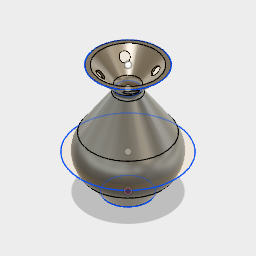
huaping (Autodesk Fusion 360 design; units mm, degrees)
Autodesk Fusion 360 part; units mm, degrees
sketch "草图1" plane through (0, 0, 0) normal (0, 1, 0) x (1, 0, 0)
  circle A0 centre (0, 0) radius 14.1421
  circle A1 through (34.6774, 0, 25) (-17.3387, 30.0315, 25) (-17.3387, -30.0315, 25)
  circle A2 through (7.0711, 0, 65) (-3.5355, 6.1237, 65) (-3.5355, -6.1237, 65)
  circle A3 through (22.3607, 0, 80) (-11.1803, 19.3649, 80) (-11.1803, -19.3649, 80)
loft "放样1" add profiles "草图1", "草图1" section 1 section 2 contours A1 in plane through (0, 25, 0) normal (0, 1, 0) makes body 1
loft "放样2" add profiles "草图1", "草图1" section 1 contours A1 in plane through (0, 25, 0) normal (0, 1, 0) section 2 contours A2 in plane through (0, 65, 0) normal (0, 1, 0) bodies 1
loft "放样3" add profiles "草图1", "草图1" section 1 contours A3 in plane through (0, 80, 0) normal (0, 1, 0) section 2 contours A2 in plane through (0, 65, 0) normal (0, 1, 0) bodies 1
sphere "球体基本要素1" add diameter 10 placed x (0, 0, -1) y (0, 1, 0) z (1, 0, 0) at (0, 72.1945, 38.3955) separate body makes body 2
move_body "MoveFace1" bodies 2 to x (1, 0, 0) y (0, 1, 0) z (0, 0, 1) at (-10.572, 0.0066, -24.9858) on bodies 2
pattern_circular "C-阵列1" count 4 over 360 about axis through (0, 25, 0) along (0, -1, 0) of bodies 2 makes body 3 at (-8.6693, 73.3831, -11.6359) makes body 4 at (11.6359, 71.0193, -8.6693) makes body 5 at (8.6693, 71.0193, 11.6359)
fillet "圆角1" radius 3 1 edges at (-6.5925, 65, -2.557) on bodies 1
fillet "圆角2" radius 20 1 edges at (-32.3307, 25, -12.5399) on bodies 1
shell "抽壳1" thickness 2 removed faces 1 at (9.2885, 80, -1.7026) on bodies 1
combine "合并1" operation cut target body 1 tool bodies 4 5 3 2
